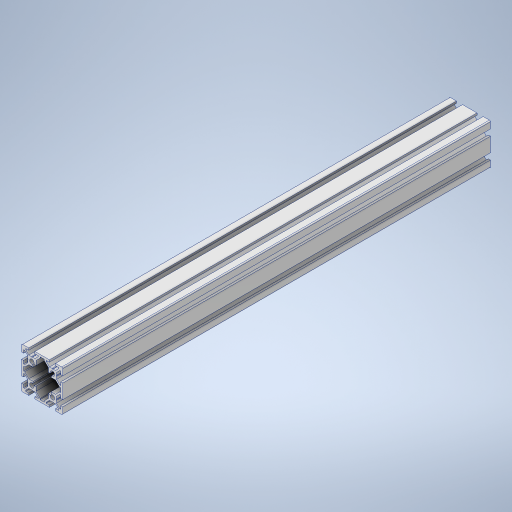
# Autodesk Inventor part: Front Base Beam
Saved by Autodesk Inventor 2024 (Build 280153000, 153)
## iProperties
Category: PARTsolutions
Company: MISUMI
Created: 2024-12-11
Part Number: Front Base Beam
Material: Aluminum 6061
Catalog Web Link: www.cadenas.de
Description: NFS5-4040, NFSB5-4040, HFS5-4040, HFSB5-4040, CAF5-4040, NFSF5-4040, HFSF5-4040, HFST5-4040, HFSY5-4040-Aluminum Frames -5 Series-2 Row Groove 40 mm Square-Specified Length
Vendor: MISUMI
Document SubType Name: Modeling
Designer: psAdmin
Manufacturer: MISUMI
Mass: 199.562 g
Surface Area: 2037.83 cm^2
Volume: 199.562 cm^3
Density: 2.7 g/cm^3
Appearance: Aluminum - Flat
PSOL_IDENT_0: {$CADENAS_DATA/23d-libs/misumi/metric/38_al_extrusions_blackets/5/hfs5_4040.prj},639 {VTYP=3D},{NB=H
PSOL_IDENT_1: FS5-4040-415},{LINA=HFS5-4040-415},{NN=NFS5-4040, NFSB5-4040, HFS5-4040, HFSB5-4040, CAF5-4040, NFSF
PSOL_IDENT_2: 5-4040, HFSF5-4040, HFST5-4040, HFSY5-4040},{DATE=31.05.2023 08:06:27},{GEOMDATE=23.09.2021 06:48:02
PSOL_IDENT_3: },{VERSION=},{LINEID=150},{WBVAR=L,ALT1,ALT2,ALT4,ALT5,CP5,DL5,DR5,ALT6,ALT9,ALT10,ALT11,HP6,NHL6,DL
PSOL_IDENT_4: 6,NHR6,DR6,ALT7,ALT8,NH9,AH,BH,CH,DH,EH,NH10,AV,BV,CV,DV,EV,NH11,AP,BP,CP,DP,EP,ALT12,ALT13,Z,NH12,X
PSOL_IDENT_5: A,XB,XC,XD,XE,NH13,YA,YB,YC,YD,YE,ALT16,HP16,DL16,DR16,ALT17,HQ17,JLP,ALT18,HQ18,KLP,ALT20},{WBNUMER
PSOL_IDENT_6: IC=L,NH9,AH,BH,CH,DH,EH,NH10,AV,BV,CV,DV,EV,NH11,AP,BP,CP,DP,EP,NH12,XA,XB,XC,XD,XE,NH13,YA,YB,YC,YD
PSOL_IDENT_7: ,YE,HQ17,JLP,HQ18,KLP}  {NB=HFS5-4040-415},{LINA=HFS5-4040-415},{KT=DUMMY},{PN=HFS5-4040-415},{TPS=H
PSOL_IDENT_8: FS5-4040},{MAT=A6N01SS-T5 Aluminum Alloy or 6005A-T5 Aluminum Alloy},{ST=Clear Anodize},{FRMW=40},{F
PSOL_IDENT_9: RMH=40},{FRD=4.2},{L=415},{MASS=1.28},{SA=472},{LX=8.89x10^4},{LY=8.89x10^4},{ALT1=},{M1=0},{DPL1=0}
PSOL_IDENT_10: ,{DPR1=0},{ALT1PN=},{ALT2=},{ALT2ALG= '','w/o End Tapping (Insert)','LHP','with LHP (Tapping on the
PSOL_IDENT_11: Left (Insert))','RHP','with RHP (Tapping on the Right (Insert))','HPW','with HPW (Tapping on Both En
PSOL_IDENT_12: ds (Insert))' },{M2=0},{DP2=0},{ALT2PN=},{ALT4=},{ALT4ALG= '', 'w/o SC (High Precision Cut)', 'SC', '
PSOL_IDENT_13: with SC (High Precision Cut)' },{ALT4PN=},{ALT5=},{ALT5ALG= '','w/o 45 Degree Cut','1','with 45 Degr
PSOL_IDENT_14: ee Cut' },{CP5=},{CP5ALG= '','N/A' },{DL5=},{DL5ALG= '','N/A' },{DR5=},{DR5ALG= '','N/A' },{FRMLALT5=
PSOL_IDENT_15: 0},{FRMRALT5=0},{ALT5PN=},{ALT6=},{ALT6ALG= '','w/o Fastening Location Wrench Access Hole Alteration
PSOL_IDENT_16: s','1','with Fastening Location Wrench Access Hole Alterations' },{ALT9=},{ALT9ALG= '','w/o Location
PSOL_IDENT_17: Specified Wrench Access Hole Alteratons (Horizontal)','1','with Location Specified Wrench Access Ho
PSOL_IDENT_18: le Alteratons (Horizontal)' },{ALT10=},{ALT10ALG= '','w/o Location Specified Wrench Access Hole Alte
PSOL_IDENT_19: ratons (Vertical)','1','with Location Specified Wrench Access Hole Alteratons (Vertical)' },{ALT11=}
PSOL_IDENT_20: ,{ALT11ALG= '','w/o Location Specified Wrench Access Hole Alteratons (Crisscross)','1','with Locatio
PSOL_IDENT_21: n Specified Wrench Access Hole Alteratons (Crisscross)' },{DD6=0.00},{DD6ALG=0},{HP6=},{HP6ALG= '','
PSOL_IDENT_22: N/A' },{NHL6=},{NHL6ALG= '','N/A' },{DL6=},{DL6ALG= '','N/A' },{NHR6=},{NHR6ALG= '','N/A' },{DR6=},{
PSOL_IDENT_23: DR6ALG= '','N/A' },{DD6PN=},{HL6=0},{HL6D=0},{HR6=0},{HR6D=0},{J6=0},{J6D=0},{K6=0},{K6D=0},{ALT7=},
PSOL_IDENT_24: {ALT7ALG= '','N/A' },{ALT8=},{ALT8ALG= '','N/A' },{ALT678PN=},{NH9=0},{NH9MAX=5},{NH9ALG=[0]},{AH=0.
PSOL_IDENT_25: 0},{AHMIN=7},{AHMAX=410},{AHALG=[0]},{BH=0.0},{BHMIN=2},{BHMAX=412},{BHALG=[0]},{CH=0.0},{CHMIN=2},{
PSOL_IDENT_26: CHMAX=414},{CHALG=[0]},{DH=0.0},{DHMIN=2},{DHMAX=416},{DHALG=[0]},{EH=0.0},{EHMIN=2},{EHMAX=408},{EH
PSOL_IDENT_27: ALG=[0]},{NH10=0},{NH10MAX=5},{NH10ALG=[0]},{AV=0.0},{AVMIN=7},{AVMAX=410},{AVALG=[0]},{BV=0.0},{BVM
PSOL_IDENT_28: IN=2},{BVMAX=412},{BVALG=[0]},{CV=0.0},{CVMIN=2},{CVMAX=414},{CVALG=[0]},{DV=0.0},{DVMIN=2},{DVMAX=4
PSOL_IDENT_29: 16},{DVALG=[0]},{EV=0.0},{EVMIN=2},{EVMAX=408},{EVALG=[0]},{NH11=0},{NH11MAX=5},{NH11ALG=[0]},{AP=0.
PSOL_IDENT_30: 0},{APMIN=7},{APMAX=410},{APALG=[0]},{BP=0.0},{BPMIN=2},{BPMAX=412},{BPALG=[0]},{CP=0.0},{CPMIN=2},{
PSOL_IDENT_31: CPMAX=414},{CPALG=[0]},{DP=0.0},{DPMIN=2},{DPMAX=416},{DPALG=[0]},{EP=0.0},{EPMIN=2},{EPMAX=408},{EP
PSOL_IDENT_32: ALG=[0]},{ALT9PN=},{ALT10PN=},{ALT11PN=},{ALT91011PN=},{ALT12=},{ALT12ALG= '','w/o Counterbore Hole
PSOL_IDENT_33: in Specified Position (Vertical)','1','with Counterbore Hole in Specified Position (Vertical)' },{AL
PSOL_IDENT_34: T13=},{ALT13ALG= '','w/o Counterbore Hole in Specified Position (Horizontal)','1','with Counterbore
PSOL_IDENT_35: Hole in Specified Position (Horizontal)' },{Z=},{ZALG= '','N/A' },{DD12=0.0},{DD112=0.0},{NH12=0},{N
PSOL_IDENT_36: H12MAX=5},{NH12ALG=[0]},{XA=0.0},{XAMIN=7},{XAMAX=410},{XAALG=[0]},{XB=0.0},{XBMIN=2},{XBMAX=412},{X
PSOL_IDENT_37: BALG=[0]},{XC=0.0},{XCMIN=2},{XCMAX=414},{XCALG=[0]},{XD=0.0},{XDMIN=2},{XDMAX=416},{XDALG=[0]},{XE=
PSOL_IDENT_38: 0.0},{XEMIN=2},{XEMAX=408},{XEALG=[0]},{NH13=0},{NH13MAX=5},{NH13ALG=[0]},{YA=0.0},{YAMIN=7},{YAMAX=
PSOL_IDENT_39: 410},{YAALG=[0]},{YB=0.0},{YBMIN=2},{YBMAX=412},{YBALG=[0]},{YC=0.0},{YCMIN=2},{YCMAX=414},{YCALG=[0
PSOL_IDENT_40: ]},{YD=0.0},{YDMIN=2},{YDMAX=416},{YDALG=[0]},{YE=0.0},{YEMIN=2},{YEMAX=408},{YEALG=[0]},{ALT12PN=},
PSOL_IDENT_41: {ALT13PN=},{ALT1213PN=},{ALT16=},{ALT16ALG= '','w/o M Type Hole Alteration','1','with M Type Hole Al
PSOL_IDENT_42: teration' },{HP16=},{HP16ALG= '','N/A' },{DL16=},{DL16ALG= '','N/A' },{DR16=},{DR16ALG= '','N/A' },{
PSOL_IDENT_43: H116=0},{D16=0.0},{ALT16PN=},{ALT17=},{ALT17ALG= '','w/o L Type Hole Alteration (Top)','1','with L T
PSOL_IDENT_44: ype Hole Alteration (Top)' },{HQ17=0},{HQ17ALG=0},{JLP=0},{JLPMIN=4.9},{JLPMAX=0},{JLPALG=[0]},{L17=
PSOL_IDENT_45: 0},{D17=0.0},{ALT17PN=},{ALT18=},{ALT18ALG= '','w/o L Type Hole Alteration (Bottom)','1','with L Typ
PSOL_IDENT_46: e Hole Alteration (Bottom)' },{HQ18=0},{HQ18ALG=0},{KLP=0},{KLPMIN=4.9},{KLPMAX=0},{KLPALG=[0]},{L18=
PSOL_IDENT_47: 0},{D18=0.0},{ALT18PN=},{ALT20=},{ALT20PN=},{ERRORALT01=OK},{ERRORALT02=OK},{ERRORALT05=OK},{ERRORAL
PSOL_IDENT_48: T06091=OK},{ERRORALT06092=OK},{ERRORALT06093=OK},{ERRORALT06094=OK},{ERRORALT06101=OK},{ERRORALT0610
PSOL_IDENT_49: 2=OK},{ERRORALT06103=OK},{ERRORALT06104=OK},{ERRORALT06111=OK},{ERRORALT06112=OK},{ERRORALT06113=OK}
PSOL_IDENT_50: ,{ERRORALT06114=OK},{ERRORALT06121=OK},{ERRORALT06122=OK},{ERRORALT06123=OK},{ERRORALT06124=OK},{ERR
PSOL_IDENT_51: ORALT06131=OK},{ERRORALT06132=OK},{ERRORALT06133=OK},{ERRORALT06134=OK},{ERRORALT0616=OK},{ERRORALT0
PSOL_IDENT_52: 6171=OK},{ERRORALT06172=OK},{ERRORALT06173=OK},{ERRORALT06181=OK},{ERRORALT06182=OK},{ERRORALT06183=
PSOL_IDENT_53: OK},{ERRORALT0911=OK},{ERRORALT0913=OK},{ERRORALT0916=OK},{ERRORALT0917=OK},{ERRORALT0918=OK},{ERROR
PSOL_IDENT_54: ALT1011=OK},{ERRORALT1012=OK},{ERRORALT1016=OK},{ERRORALT1017=OK},{ERRORALT1018=OK},{ERRORALT1112=OK
PSOL_IDENT_55: },{ERRORALT1113=OK},{ERRORALT1116=OK},{ERRORALT1117=OK},{ERRORALT1118=OK},{ERRORALT1216=OK},{ERRORAL
PSOL_IDENT_56: T1217=OK},{ERRORALT1218=OK},{ERRORALT1316=OK},{ERRORALT1317=OK},{ERRORALT1318=OK},{ERRORALT1617=OK},
PSOL_IDENT_57: {ERRORALT1618=OK},{ERRORPN=},{TFW=0},{IDM1=4.134},{COLOR=}
NB: HFS5-4040-415
NN: NFS5-4040, NFSB5-4040, HFS5-4040, HFSB5-4040, CAF5-4040, NFSF5-4040, HFSF5-4040, HFST5-4040, HFSY5-4040
NT: Aluminum Frames -5 Series-2 Row Groove 40 mm Square-Specified Length
NBSYN: $PN.
LINA: HFS5-4040-415
CATALOG: Misumi
PN: HFS5-4040-415
TPS: HFS5-4040
MAT: A6N01SS-T5 Aluminum Alloy or 6005A-T5 Aluminum Alloy
ST: Clear Anodize
L: 415
MASS: 1.28
SA: 472
LX: 8.89x10^4
LY: 8.89x10^4
ALT1: w/o End Tapping
M1: 0
DPL1: 0
DPR1: 0
ALT2: w/o End Tapping (Insert)
M2: 0
DP2: 0
ALT4: w/o SC (High Precision Cut)
ALT5: w/o 45 Degree Cut
CP5: N/A
DL5: N/A
DR5: N/A
ALT6: w/o Fastening Location Wrench Access Hole Alterations
ALT9: w/o Location Specified Wrench Access Hole Alteratons (Horizontal)
ALT10: w/o Location Specified Wrench Access Hole Alteratons (Vertical)
ALT11: w/o Location Specified Wrench Access Hole Alteratons (Crisscross)
DD6: 0
HP6: N/A
NHL6: N/A
DL6: N/A
NHR6: N/A
DR6: N/A
HL6D: 0
HR6D: 0
J6D: 0
K6D: 0
ALT7: N/A
ALT8: N/A
NH9: 0
AH: 0
BH: 0
CH: 0
DH: 0
EH: 0
NH10: 0
AV: 0
BV: 0
CV: 0
DV: 0
EV: 0
NH11: 0
AP: 0
BP: 0
CP: 0
DP: 0
EP: 0
ALT12: w/o Counterbore Hole in Specified Position (Vertical)
ALT13: w/o Counterbore Hole in Specified Position (Horizontal)
Z: N/A
DD12: 0
DD112: 0
NH12: 0
XA: 0
XB: 0
XC: 0
XD: 0
XE: 0
NH13: 0
YA: 0
YB: 0
YC: 0
YD: 0
YE: 0
ALT16: w/o M Type Hole Alteration
HP16: N/A
DL16: N/A
DR16: N/A
H116: 0
D16: 0
ALT17: w/o L Type Hole Alteration (Top)
HQ17: 0
JLP: 0
D17: 0
ALT18: w/o L Type Hole Alteration (Bottom)
HQ18: 0
KLP: 0
D18: 0
ALT20: w/o CW (End Face C Chamfering)
SUPPLIER: MISUMI
ARTICLENO: HFS5-4040-415
BOMINFO: HFS5-4040-415
CREATOR: CADENAS GmbH
Title: HFS5-4040-415
Author: Cadenas PARTsolutions
Comments: Aluminum Frames -5 Series-2 Row Groove 40 mm Square-Specified Length
Autodesk Inventor part; units mm, degrees
sketch "Sketch_1" plane through (0, 0, 0) normal (0, 0, 1) x (1, 0, 0)
  line L0 (-20, -7) -> (-18, -7)
  line L1 (-18, -7) -> (-18, -4)
  line L2 (-18, -4) -> (-17.0607, -4)
  line L3 (-17.0607, -4) -> (-14, -7.0607)
  line L4 (-14, -7.0607) -> (-14, -9.4804)
  line L5 (-14, -9.4804) -> (-13.7, -10)
  line L6 (-13.7, -10) -> (-14, -10.5196)
  line L7 (-14, -10.5196) -> (-14, -12.9393)
  line L8 (-14, -12.9393) -> (-17.0607, -16)
  line L9 (-17.0607, -16) -> (-18, -16)
  line L10 (-18, -16) -> (-18, -13)
  line L11 (-18, -13) -> (-20, -13)
  line L12 (-20, -13) -> (-20, -19)
  arc A0 (-20, -19) -> (-19, -20) centre (-19, -19) ccw
  line L13 (-19, -20) -> (-13, -20)
  line L14 (-13, -20) -> (-13, -18)
  line L15 (-13, -18) -> (-16, -18)
  line L16 (-16, -18) -> (-16, -17.0607)
  line L17 (-16, -17.0607) -> (-12.9393, -14)
  line L18 (-12.9393, -14) -> (-10.5196, -14)
  line L19 (-10.5196, -14) -> (-10, -13.7)
  line L20 (-10, -13.7) -> (-9.4804, -14)
  line L21 (-9.4804, -14) -> (-7.0607, -14)
  line L22 (-7.0607, -14) -> (-4, -17.0607)
  line L23 (-4, -17.0607) -> (-4, -18)
  line L24 (-4, -18) -> (-7, -18)
  line L25 (-7, -18) -> (-7, -20)
  line L26 (-7, -20) -> (7, -20)
  line L27 (7, -20) -> (7, -18)
  line L28 (7, -18) -> (4, -18)
  line L29 (4, -18) -> (4, -17.0607)
  line L30 (4, -17.0607) -> (7.0607, -14)
  line L31 (7.0607, -14) -> (9.4804, -14)
  line L32 (9.4804, -14) -> (10, -13.7)
  line L33 (10, -13.7) -> (10.5196, -14)
  line L34 (10.5196, -14) -> (12.9393, -14)
  line L35 (12.9393, -14) -> (16, -17.0607)
  line L36 (16, -17.0607) -> (16, -18)
  line L37 (16, -18) -> (13, -18)
  line L38 (13, -18) -> (13, -20)
  line L39 (13, -20) -> (19, -20)
  arc A1 (19, -20) -> (20, -19) centre (19, -19) ccw
  line L40 (20, -19) -> (20, -13)
  line L41 (20, -13) -> (18, -13)
  line L42 (18, -13) -> (18, -16)
  line L43 (18, -16) -> (17.0607, -16)
  line L44 (17.0607, -16) -> (14, -12.9393)
  line L45 (14, -12.9393) -> (14, -10.5196)
  line L46 (14, -10.5196) -> (13.7, -10)
  line L47 (13.7, -10) -> (14, -9.4804)
  line L48 (14, -9.4804) -> (14, -7.0607)
  line L49 (14, -7.0607) -> (17.0607, -4)
  line L50 (17.0607, -4) -> (18, -4)
  line L51 (18, -4) -> (18, -7)
  line L52 (18, -7) -> (20, -7)
  line L53 (20, -7) -> (20, 7)
  line L54 (20, 7) -> (18, 7)
  line L55 (18, 7) -> (18, 4)
  line L56 (18, 4) -> (17.0607, 4)
  line L57 (17.0607, 4) -> (14, 7.0607)
  line L58 (14, 7.0607) -> (14, 9.4804)
  line L59 (14, 9.4804) -> (13.7, 10)
  line L60 (13.7, 10) -> (14, 10.5196)
  line L61 (14, 10.5196) -> (14, 12.9393)
  line L62 (14, 12.9393) -> (17.0607, 16)
  line L63 (17.0607, 16) -> (18, 16)
  line L64 (18, 16) -> (18, 13)
  line L65 (18, 13) -> (20, 13)
  line L66 (20, 13) -> (20, 19)
  arc A2 (20, 19) -> (19, 20) centre (19, 19) ccw
  line L67 (19, 20) -> (13, 20)
  line L68 (13, 20) -> (13, 18)
  line L69 (13, 18) -> (16, 18)
  line L70 (16, 18) -> (16, 17.0607)
  line L71 (16, 17.0607) -> (12.9393, 14)
  line L72 (12.9393, 14) -> (10.5196, 14)
  line L73 (10.5196, 14) -> (10, 13.7)
  line L74 (10, 13.7) -> (9.4804, 14)
  line L75 (9.4804, 14) -> (7.0607, 14)
  line L76 (7.0607, 14) -> (4, 17.0607)
  line L77 (4, 17.0607) -> (4, 18)
  line L78 (4, 18) -> (7, 18)
  line L79 (7, 18) -> (7, 20)
  line L80 (7, 20) -> (-7, 20)
  line L81 (-7, 20) -> (-7, 18)
  line L82 (-7, 18) -> (-4, 18)
  line L83 (-4, 18) -> (-4, 17.0607)
  line L84 (-4, 17.0607) -> (-7.0607, 14)
  line L85 (-7.0607, 14) -> (-9.4804, 14)
  line L86 (-9.4804, 14) -> (-10, 13.7)
  line L87 (-10, 13.7) -> (-10.5196, 14)
  line L88 (-10.5196, 14) -> (-12.9393, 14)
  line L89 (-12.9393, 14) -> (-16, 17.0607)
  line L90 (-16, 17.0607) -> (-16, 18)
  line L91 (-16, 18) -> (-13, 18)
  line L92 (-13, 18) -> (-13, 20)
  line L93 (-13, 20) -> (-19, 20)
  arc A3 (-19, 20) -> (-20, 19) centre (-19, 19) ccw
  line L94 (-20, 19) -> (-20, 13)
  line L95 (-20, 13) -> (-18, 13)
  line L96 (-18, 13) -> (-18, 16)
  line L97 (-18, 16) -> (-17.0607, 16)
  line L98 (-17.0607, 16) -> (-14, 12.9393)
  line L99 (-14, 12.9393) -> (-14, 10.5196)
  line L100 (-14, 10.5196) -> (-13.7, 10)
  line L101 (-13.7, 10) -> (-14, 9.4804)
  line L102 (-14, 9.4804) -> (-14, 7.0607)
  line L103 (-14, 7.0607) -> (-17.0607, 4)
  line L104 (-17.0607, 4) -> (-18, 4)
  line L105 (-18, 4) -> (-18, 7)
  line L106 (-18, 7) -> (-20, 7)
  line L107 (-20, 7) -> (-20, -7)
  constraints: 216 end point, 8 point on circle, 4 centre point
extrude "Extrusion1" add sketch "Sketch_1" against normal blind 415
sketch "Sketch_130" plane through (0, 0, 0) normal (0, 0, 1) x (1, 0, 0)
  line L0 (-18, 2) -> (-18, -2)
  line L1 (-18, -2) -> (-16.9393, -2)
  line L2 (-16.9393, -2) -> (-12.9393, -6)
  line L3 (-12.9393, -6) -> (-8.6667, -6)
  line L4 (-8.6667, -6) -> (-9.3359, -8.0078)
  arc A0 (-9.3359, -8.0078) -> (-8.0078, -9.3359) centre (-10, -10) ccw
  line L5 (-8.0078, -9.3359) -> (-6, -8.6667)
  line L6 (-6, -8.6667) -> (-6, -12.9393)
  line L7 (-6, -12.9393) -> (-2, -16.9393)
  line L8 (-2, -16.9393) -> (-2, -18)
  line L9 (-2, -18) -> (2, -18)
  line L10 (2, -18) -> (2, -16.9393)
  line L11 (2, -16.9393) -> (6, -12.9393)
  line L12 (6, -12.9393) -> (6, -8.6667)
  line L13 (6, -8.6667) -> (8.0078, -9.3359)
  arc A1 (8.0078, -9.3359) -> (9.3359, -8.0078) centre (10, -10) ccw
  line L14 (9.3359, -8.0078) -> (8.6667, -6)
  line L15 (8.6667, -6) -> (12.9393, -6)
  line L16 (12.9393, -6) -> (16.9393, -2)
  line L17 (16.9393, -2) -> (18, -2)
  line L18 (18, -2) -> (18, 2)
  line L19 (18, 2) -> (16.9393, 2)
  line L20 (16.9393, 2) -> (12.9393, 6)
  line L21 (12.9393, 6) -> (8.6667, 6)
  line L22 (8.6667, 6) -> (9.3359, 8.0078)
  arc A2 (9.3359, 8.0078) -> (8.0078, 9.3359) centre (10, 10) ccw
  line L23 (8.0078, 9.3359) -> (6, 8.6667)
  line L24 (6, 8.6667) -> (6, 12.9393)
  line L25 (6, 12.9393) -> (2, 16.9393)
  line L26 (2, 16.9393) -> (2, 18)
  line L27 (2, 18) -> (-2, 18)
  line L28 (-2, 18) -> (-2, 16.9393)
  line L29 (-2, 16.9393) -> (-6, 12.9393)
  line L30 (-6, 12.9393) -> (-6, 8.6667)
  line L31 (-6, 8.6667) -> (-8.0078, 9.3359)
  arc A3 (-8.0078, 9.3359) -> (-9.3359, 8.0078) centre (-10, 10) ccw
  line L32 (-9.3359, 8.0078) -> (-8.6667, 6)
  line L33 (-8.6667, 6) -> (-12.9393, 6)
  line L34 (-12.9393, 6) -> (-16.9393, 2)
  line L35 (-16.9393, 2) -> (-18, 2)
  constraints: 72 end point, 10 horizontal, 10 vertical, 8 point on circle, 4 centre point, 64 other
extrude "Extrusion2" cut sketch "Sketch_130" against normal blind 415
ref_plane "C1_XY" through (0, 0, 0) normal (0, 0, 1) x (1, 0, 0)
ref_plane "C1_YZ" through (0, 0, 0) normal (1, 0, 0) x (0, 1, 0)
ref_plane "C1_ZX" through (0, 0, 0) normal (0, 1, 0) x (0, 0, 1)
ref_plane "to_frame_cap1_XY" through (0, 0, 0) normal (0, 0, 1) x (1, 0, 0)
ref_plane "to_frame_cap1_YZ" through (0, 0, 0) normal (1, 0, 0) x (0, 1, 0)
ref_plane "to_frame_cap1_ZX" through (0, 0, 0) normal (0, 1, 0) x (0, 0, 1)
ref_plane "to_frame_cap2_XY" through (0, 0, -415) normal (0, 0, -1) x (1, 0, 0)
ref_plane "to_frame_cap2_YZ" through (0, 0, -415) normal (1, 0, 0) x (0, -1, 0)
ref_plane "to_frame_cap2_ZX" through (0, 0, -415) normal (0, -1, 0) x (0, 0, -1)
thread "Thread1" size "M5x0.8" class "6H" standard "ANSI Metric M Profile" length 10
thread "Thread2" size "M5x0.8" class "6H" standard "ANSI Metric M Profile" length 10
thread "Thread3" size "M5x0.8" class "6H" standard "ANSI Metric M Profile" length 10
thread "Thread4" size "M5x0.8" class "6H" standard "ANSI Metric M Profile" length 10
thread "Thread5" size "M5x0.8" class "6H" standard "ANSI Metric M Profile" length 10
thread "Thread6" size "M5x0.8" class "6H" standard "ANSI Metric M Profile" length 10
thread "Thread7" size "M5x0.8" class "6H" standard "ANSI Metric M Profile" length 10
thread "Thread8" size "M5x0.8" class "6H" standard "ANSI Metric M Profile" length 10
body "Solid1"
